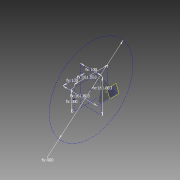
# Autodesk Inventor part: Frame
Saved by Autodesk Inventor 2014 (Build 180170000, 170)
## iProperties
Created: 2016-01-26
Part Number: Frame
Material: Generic
Document SubType Name: Modeling
Designer: Justin B
Density: 1 g/cm^3
Appearance: Default
Author: Justin B
Autodesk Inventor part; units mm, degrees
ref_plane "YZ Plane" through (0, 0, 0) normal (1, 0, 0) x (0, 1, 0)
ref_plane "XZ Plane" through (0, 0, 0) normal (0, 1, 0) x (-1, 0, 0)
ref_plane "XY Plane" through (0, 0, 0) normal (0, 0, 1) x (1, 0, 0)
sketch "Sketch1" plane through (0, 0, 0) normal (0, 1, 0) x (-1, 0, 0)
  line L0 (-80.9017, 50) -> (80.9017, 50) construction
  line L1 (80.9017, 50) -> (80.9017, -50) construction
  line L2 (80.9017, -50) -> (-80.9017, -50) construction
  line L3 (-80.9017, -50) -> (-80.9017, 50) construction
  point P0 (0, 0)
  point P1 (0, 50)
  point P2 (80.9017, 0)
  dimension "d1" = 100
  dimension "d6" = 161.8034
  constraints: 8 end point, 2 midpoint, 2 parallel, 1 horizontal, 1 horizontal alignment, 1 perpendicular, 1 vertical alignment
  measures "d1" distance of L0.end L1.end
  measures "d6" distance of L0.start L0.end
sketch "Sketch2" plane through (0, 0, 0) normal (0, 0, 1) x (1, 0, 0)
  line L0 (-50, 80.9017) -> (50, 80.9017) construction
  line L1 (50, 80.9017) -> (50, -80.9017) construction
  line L2 (50, -80.9017) -> (-50, -80.9017) construction
  line L3 (-50, -80.9017) -> (-50, 80.9017) construction
  point P0 (0, 0)
  point P1 (0, 80.9017)
  point P2 (50, 0)
  dimension "d3" = 161.8034
  dimension "d7" = 100
  constraints: 8 end point, 2 midpoint, 2 parallel, 1 horizontal, 1 horizontal alignment, 1 perpendicular, 1 vertical alignment
  measures "d3" distance of L0.end L1.end
  measures "d7" distance of L0.start L0.end
sketch "Sketch3" plane through (0, 0, 0) normal (1, 0, 0) x (0, 1, 0)
  line L0 (-50, 80.9017) -> (50, 80.9017) construction
  line L1 (50, 80.9017) -> (50, -80.9017) construction
  line L2 (50, -80.9017) -> (-50, -80.9017) construction
  line L3 (-50, -80.9017) -> (-50, 80.9017) construction
  point P0 (0, 0)
  point P1 (50, 0)
  point P2 (0, 80.9017)
  dimension "d4" = 161.8034
  dimension "d5" = 100
  constraints: 8 end point, 2 midpoint, 2 parallel, 1 horizontal, 1 horizontal alignment, 1 perpendicular, 1 vertical alignment
  measures "d4" distance of L0.end L1.end
  measures "d5" distance of L0.start L0.end
sketch "Sketch7" plane through (0, 0, 0) normal (1, 0, 0) x (0, 1, 0)
  circle A0 centre (0, 0) radius 200 construction
  dimension "BallDiameter" = 400
  constraints: 1 centre point, 1 coincident
  measures "BallDiameter" diameter of A0
ref_plane "Work Plane2" through (80.9017, 0, -50) normal (-0.9341724, -0.3568221, 0) x (0, 0, 1)
sketch "Sketch8" plane through (80.9017, 0, -50) normal (-0.9341724, -0.3568221, 0) x (0, 0, 1)
  line L0 (50, 86.6025) -> (0, 0) construction
  line L1 (0, 0) -> (100, 0) construction
  line L2 (100, 0) -> (50, 86.6025) construction
  line L3 (3.4641, 2) -> (50, 82.6025)
  line L4 (50, 82.6025) -> (96.5359, 2)
  line L5 (96.5359, 2) -> (3.4641, 2)
  point P0 (50, 28.8675)
  dimension "d21" = 2
  dimension "d22" = 2
  dimension "d23" = 2
  constraints: 12 end point, 2 equal length, 2 horizontal
  measures "d21" distance between parallel lines of L2 L4
  measures "d22" distance between parallel lines of L1 L5
  measures "d23" distance between parallel lines of L0 L3
extrude "Extrusion3" add sketch "Sketch8" along normal blind 2
fillet "Fillet1" radius 10 3 edges at (79.2539, 1.5115, -46.5359) (79.2539, 1.5115, 46.5359) (50.4931, 76.8082, 0)
sketch "Sketch11" plane through (80.9017, 0, -50) normal (0.9341724, 0.3568221, 0) x (0, 0, -1)
  circle A0 centre (-50, 28.8675) radius 5
  dimension "d34" = 10
  constraints: 1 centre point, 1 coincident
  measures "d34" diameter of A0
hole "Hole2" at (70.6011, 26.9672, 0) direction (-0.9341724, -0.3568221, 0) diameter 10 end through all
sketch "Sketch10" plane through (80.9017, 0, -50) normal (0.9341724, 0.3568221, 0) x (0, 0, -1)
  arc A0 (-41.3397, 67.6025) -> (-58.6603, 67.6025) centre (-50, 62.6025) ccw projected
  circle A1 centre (-50, 62.6025) radius 1.5
  point P0 (-50, 28.8675)
  dimension "d25" = 3
  constraints: 1 centre point, 1 coincident
  measures "d25" diameter of A1
hole "Hole1" at (58.5637, 58.4816, 0) direction (-0.9341724, -0.3568221, 0) diameter 3 end through all
pattern_circular "Circular Pattern1" count 3 over 360 about axis through (-28.8274, -11.0111, 0) along (0.9341724, 0.3568221, 0) of "Hole1"
equation "\"d1\" = IcoLen"
equation "\"d6\" = IcoWidth"
equation "\"d3\" = IcoWidth"
equation "\"d7\" = IcoLen"
equation "\"d4\" = IcoWidth"
equation "\"d5\" = IcoLen"
equation "\"BallDiameter\" = 2 * BallRadius"
equation "\"IcoLen\" = 100"
equation "\"IcoWidth\" = 1.61803 * IcoLen"
equation "\"BallRadius\" = 200"
body "Solid2"
